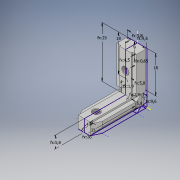
# Autodesk Inventor part: BT000_trajan20_21
Saved by Autodesk Inventor 2022.2 (Build 262287000, 287)
## iProperties
Company: HTBLA Kaindorf
RuleStatus: InUse
Created: 2022-07-23
Part Number: BT000_trajan20_21
Project: Innenwinkel
Material: Generisch
Description: MS
Document SubType Name: Modeling
Designer: trajan20
Density: 1 g/cm^3
Appearance: Vorgabe
Mass: 2.03731 g
Surface Area: 14.8059 cm^2
Volume: 2.03731 cm^3
AfterDocNew0: iProperties-Editor_aufrufen
Author: jan
Keywords: 2021
Autodesk Inventor part; units mm, degrees
ref_plane "YZ Plane" through (0, 0, 0) normal (1, 0, 0) x (0, 1, 0)
ref_plane "XZ Plane" through (0, 0, 0) normal (0, 1, 0) x (-1, 0, 0)
ref_plane "XY Plane" through (0, 0, 0) normal (0, 0, 1) x (1, 0, 0)
sketch "Skizze3" plane through (0, 0, 0) normal (1, 0, 0) x (0, 1, 0)
  line L0 (4.8, 5) -> (-4.8, 5)
  line L1 (2.9, 5) -> (2.9, 25)
  line L2 (2.9, 25) -> (-2.9, 25)
  line L3 (-2.9, 25) -> (-2.9, 5)
  line L4 (-2.9, 25) -> (-4.8, 25)
  line L5 (-4.8, 25) -> (-4.8, 7)
  line L6 (-4.8, 7) -> (-2.9, 7)
  line L7 (2.9, 7) -> (4.8, 7)
  line L8 (4.8, 7) -> (4.8, 25)
  line L9 (4.8, 25) -> (2.9, 25)
  line L10 (0, -5) -> (0, 30) projected
  line L11 (4.8, 5) -> (4.8, 2.5)
  line L12 (-2.9, 0) -> (-4.8, 2.5)
  line L13 (-4.8, 2.5) -> (-4.8, 5)
  line L14 (4.8, 2.5) -> (2.9, 0)
  line L15 (2.9, 0) -> (-2.9, 0)
  line L16 (-6.72, 0) -> (6.72, 0) projected
  line L17 (-2.9, 0) -> (-4.8, 0)
  line L18 (-4.8, 2.5) -> (-4.8, 0)
  line L19 (4.8, 2.5) -> (4.8, 0)
  line L20 (4.8, 0) -> (2.9, 0)
  line L21 (4.8, 5) -> (4.8, 7)
  line L22 (-4.8, 5) -> (-4.8, 7)
  point P0 (0, 0)
  point P1 (0, 25)
  point P2 (0, 5)
  point P3 (0, 0)
  point P4 (0, 16)
  dimension "d5" = 9.6
  dimension "d6" = 5.8
  dimension "d7" = 1.9
  dimension "d9" = 18
  dimension "d10" = 18
  dimension "d12" = 9.6
  dimension "d14" = 2.9
  dimension "d15" = 2.5
  dimension "d16" = 5.8
  dimension "d17" = 2.5
  dimension "d18" = 5
  dimension "d19" = 25
  dimension "d40" = 9
  constraints: 42 end point, 10 point on line, 7 perpendicular, 4 midpoint, 3 horizontal, 2 collinear, 2 vertical, 1 parallel
  measures "d5" distance between parallel lines of L8 L5
  measures "d6" distance between parallel lines of L1 L3
  measures "d7" distance between parallel lines of L5 L3
  measures "d9" distance between parallel lines of L4 L6
  measures "d10" distance between parallel lines of L9 L7
  measures "d12" distance of L0.start L0.end
  measures "d14" distance from line of L10 L12.start
  measures "d15" distance of L12.end L0.end
  measures "d16" distance of L14.end L12.start
  measures "d17" distance of L0.start L11.end
  measures "d18" distance between parallel lines of L16 L0
  measures "d19" distance between parallel lines of L2 L16
  measures "d40" distance from line of L2 point (0, 16)
sketch "Skizze4" plane through (0, 0, 0) normal (0, 1, 0) x (-1, 0, 0)
  line L0 (0, 25) -> (0, 7) projected
  line L1 (0, 2.5) -> (0, 5) projected
  line L2 (0, 0) -> (0, 25)
  line L3 (0, 25) -> (-5.8, 25)
  line L4 (-5.8, 25) -> (-5.8, 5.8)
  line L5 (-5.8, 5.8) -> (-26, 5.8)
  line L6 (-26, 5.8) -> (-26, 0)
  line L7 (-26, 0) -> (0, 0)
  line L8 (-0.65, 25) -> (-0.65, 7)
  line L9 (-0.65, 7) -> (-5.15, 7)
  line L10 (-5.15, 7) -> (-5.15, 25)
  line L11 (-1, 0) -> (-1, 5)
  line L12 (-1, 5) -> (-26, 5)
  line L13 (-1, 0) -> (-5, 2.5)
  line L14 (-5, 2.5) -> (-22, 2.5)
  line L15 (-22, 2.5) -> (-26, 0)
  line L16 (-22, 2.5) -> (-22, 5)
  line L17 (-5, 2.5) -> (-5, 5)
  point P0 (0, 0)
  point P1 (0, 0)
  dimension "d20" = 5.8
  dimension "d21" = 4.5
  dimension "d22" = 0.65
  dimension "d23" = 26
  dimension "d24" = 5.8
  dimension "d25" = 25
  dimension "d26" = 4
  dimension "d27" = 4
  constraints: 32 end point, 11 perpendicular, 9 point on line, 1 collinear, 1 horizontal, 1 vertical
  measures "d20" distance between parallel lines of L0 L4
  measures "d21" distance between parallel lines of L10 L8
  measures "d22" distance between parallel lines of L0 L8
  measures "d23" distance between parallel lines of L6 L2
  measures "d24" distance between parallel lines of L7 L5
  measures "d25" distance between parallel lines of L6 L11
  measures "d26" distance between parallel lines of L11 L17
  measures "d27" distance between parallel lines of L6 L16
sketch "Skizze5" plane through (0, 0, 0) normal (0, 0, 1) x (1, 0, 0)
  line L0 (5.15, 4.8) -> (0.65, 4.8)
  line L1 (0.65, 4.8) -> (0.65, 2.9)
  line L2 (0.65, 2.9) -> (0, 2.9)
  line L3 (0, 2.9) -> (0, -2.9)
  line L4 (0, -2.9) -> (0.65, -2.9)
  line L5 (0.65, -2.9) -> (0.65, -4.8)
  line L6 (0.65, -4.8) -> (5.15, -4.8)
  line L7 (5.15, -4.8) -> (5.15, -2.9)
  line L8 (5.15, -2.9) -> (5.8, -2.9)
  line L9 (5.8, -2.9) -> (5.8, 2.9)
  line L10 (5.8, 2.9) -> (5.15, 2.9)
  line L11 (5.15, 4.8) -> (5.15, 2.9)
  line L12 (0, -2.9) -> (26, -2.9)
  line L13 (26, -2.9) -> (26, 2.9)
  line L14 (26, 2.9) -> (0, 2.9)
  line L15 (26, -2.9) -> (22, -4.8)
  line L16 (22, -4.8) -> (5, -4.8)
  line L17 (1, -2.9) -> (5, -4.8)
  line L18 (22, -7.8717) -> (22, 8.228) construction
  line L19 (5, -6.3703) -> (5, 8.228) construction
  line L20 (1, -9.3021) -> (1, 6.7781) construction
  line L21 (26, 2.9) -> (22, 4.8)
  line L22 (5, 4.8) -> (1, 2.9)
  line L23 (5, 4.8) -> (22, 4.8)
  line L24 (26, 0) -> (0, 0) projected
  point P0 (5.8, 0)
  point P1 (5.15, 0)
  point P2 (0.65, 0)
  point P3 (0, 4.8)
  point P4 (0, -4.8)
  point P5 (1, 0)
  point P6 (1, 0)
  point P7 (1, 0)
  point P8 (5, 0)
  point P9 (5, 0)
  point P10 (5, 0)
  point P11 (22, 0)
  point P12 (22, 0)
  point P13 (22, 0)
  point P14 (26, 0)
  point P15 (26, 0)
  point P16 (20, 0)
  dimension "d41" = 6
  constraints: 48 end point, 25 point on line, 10 perpendicular, 2 horizontal, 2 midpoint, 2 parallel, 1 coincident, 1 vertical, 2 other
  measures "d41" distance from line of L13 point (20, 0)
extrude "Extrusion6" add sketch "Skizze5" along normal blind 25 contours L11 L14 L22 L0 | L22 L14 L1 L0 | L10 L9 L24 L3 L2 L14 | L9 L8 L12 L4 L3 L24 | L7 L6 L17 L12 | L17 L6 L5 L12
extrude "Extrusion7" cut sketch "Skizze3" along normal through all contours L0 L1 L7 L21 | L0 L22 L6 L3
extrude "Extrusion3" add sketch "Skizze5" along normal blind 5 separate body contours L11 L14 L22 L0 | L23 L21 L14 L10 L11 | L10 L9 L24 L3 L2 L14 | L14 L13 L24 L9 | L24 L13 L12 L9 | L9 L8 L12 L4 L3 L24 | L12 L15 L16 L7 L8 | L7 L6 L17 L12
extrude "Extrusion5" add sketch "Skizze5" along normal blind 5.8 contours L14 L13 L24 L9 | L24 L13 L12 L9
extrude "Extrusion4" cut sketch "Skizze3" along normal through all contours L19 L16 L14 | L16 L18 L12
extrude "Extrusion8" cut sketch "Skizze5" along normal up to surface (5 mm away) contours L22 L14 L1 L0 | L17 L6 L5 L12
hole "Bohrung1" at (20, 0, 0) direction (0, 0, 1) diameter 3.242 end through all thread size "M4x0.7" class "6H" standard "ISO Metric profile"
hole "Bohrung2" at (0, 0, 16) direction (1, 0, 0) diameter 3.242 end through all thread size "M4x0.7" class "6H" standard "ISO Metric profile"
chamfer "Fase1" distance 0.2 angle 45 4 edges at (0, 0, 14.379) (5.8, 0, 14.379) (20, -1.621, 5.8) (20, -1.621, 0)
equation "\"d5\" = H2"
equation "\"d6\" = H1"
equation "\"d7\" = -0.5 * d6 + 0.5 * d5"
equation "\"d12\" = d5"
equation "\"d14\" = 0.5 * d16"
equation "\"d19\" = L2"
equation "\"d20\" = G2"
equation "\"d21\" = G1"
equation "\"d22\" = -0.5 * d21 + 0.5 * d20"
equation "\"d23\" = L1"
equation "\"d24\" = G2"
equation "\"d34\" = L2"
equation "\"d32\" = d24"
equation "\"d38\" = L2"
equation "\"L1\" = 26"
equation "\"L2\" = 25"
equation "\"H1\" = 5.8"
equation "\"H2\" = 9.6"
equation "\"G1\" = 4.5"
equation "\"G2\" = 5.8"
equation "\"M\" = 4"
